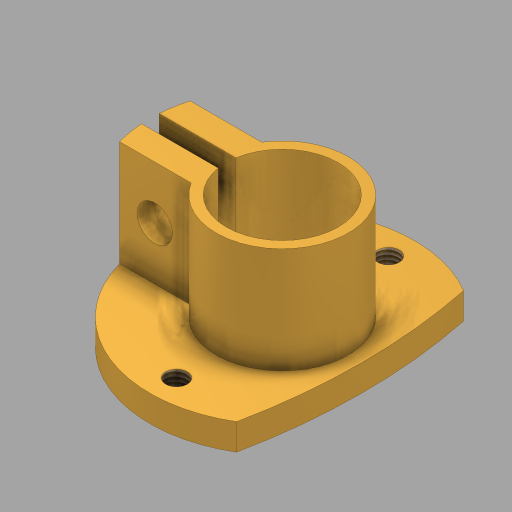
# Autodesk Inventor part: BaffleClampWithScrew
Saved by Autodesk Inventor 2024 (Build 280153020, 153B)
## iProperties
Created: 2023-10-26
Part Number: BaffleClampWithScrew
Material: Brass, Soft Yellow
Document SubType Name: Modeling
Designer: schanen
Density: 8.47 g/cm^3
Appearance: Brass - Satin
Mass: 5.52616 g
Surface Area: 9.72882 cm^2
Volume: 0.652439 cm^3
Author: schanen
Autodesk Inventor part; units mm, degrees
ref_plane "YZ Plane" through (0, 0, 0) normal (1, 0, 0) x (0, 1, 0)
ref_plane "XZ Plane" through (0, 0, 0) normal (0, 1, 0) x (-1, 0, 0)
ref_plane "XY Plane" through (0, 0, 0) normal (0, 0, 1) x (1, 0, 0)
sketch "Sketch1" plane through (0, 0, 0) normal (0, 0, 1) x (1, 0, 0)
  line L0 (-15, 0) -> (-6.35, 0)
  line L1 (-6.35, 0) -> (-6.35, 15)
  line L2 (-6.35, 15) -> (-7.5, 15)
  line L3 (-7.5, 15) -> (-7.5, 3)
  line L4 (-7.5, 3) -> (-15, 3)
  line L5 (-15, 3) -> (-15, 0)
  line L6 (0, -3) -> (0, 18) projected
  point P0 (0, 0)
  dimension "d0" = 3
  dimension "d2" = 15
  dimension "d3" = 6.35
  dimension "d4" = 15
  dimension "d17" = 7.5
  dimension "d18" = 1.15
  constraints: 12 end point, 4 perpendicular, 1 horizontal, 1 horizontal alignment, 1 parallel
  measures "d0" distance of L4.end L0.start
  measures "d2" distance of L0.end L1.end
  measures "d3" distance from line of point (0, 0) L1
  measures "d4" distance from line of point (0, 0) L5
  measures "d17" distance between parallel lines of L6 L3
  measures "d18" distance between parallel lines of L1 L3
revolve "Revolution1" add sketch "Sketch1" angle 360 about axis through (0, -10, 0) along (0, 1, 0)
sketch "Sketch2" plane through (0, 3, 0) normal (0, 1, 0) x (1, 0, 0)
  point P0 (0, 0)
  point P1 (0.0472, 12)
  point P2 (0, -12)
  dimension "d6" = 12
  dimension "d22" = 12
  measures "d6" vertical distance of point (0, 0) point (0.047, 12)
  measures "d22" distance of point (0, 0) point (0, -12)
hole "Hole1" at (0.0472, 3, -12) at (0, 3, 12) direction (0, -1, 0) diameter 2.459 end through all thread size "M3x0.5" class "6H" standard "ISO Metric profile"
sketch "Sketch4" plane through (0, 3, 0) normal (0, 1, 0) x (1, 0, 0)
  circle A0 centre (0, 0) radius 15 projected
  circle A1 centre (0, 0) radius 7.5 projected
  circle A2 centre (-55, 0) radius 64
  point P0 (7.6909, 12.8783)
  point P1 (7.5, 0)
  point P2 (7.6909, -12.8783)
  dimension "d23" = 128
  dimension "d24" = 55
  constraints: 1 centre point, 1 horizontal alignment
  measures "d23" diameter of A2
  measures "d24" distance of A2.centre point (0, 0)
extrude "Extrusion2" cut sketch "Sketch4" against normal through all contours A0 A2 picked at (10.8452, -2.4648)
sketch "Sketch6" plane through (0, 3, 0) normal (0, 1, 0) x (1, 0, 0)
  arc A0 (7.6909, 12.8783) -> (7.6909, -12.8783) centre (0, 0) ccw projected
  circle A1 centre (0, 0) radius 7.5 projected
  line L0 (-6.3443, 4) -> (-15, 4)
  line L1 (-15, 4) -> (-15, -4)
  line L2 (-15, -4) -> (-6.3443, -4)
  line L3 (-6.3443, -4) -> (-6.3443, 4)
  point P0 (-14.4568, -4)
  point P1 (-6.3443, -4)
  point P2 (-14.4568, 4)
  dimension "d32" = 4
  dimension "d33" = 4
  constraints: 8 end point, 2 parallel, 1 horizontal, 1 perpendicular, 2 other
  measures "d32" distance from line of point (0, 0) L2
  measures "d33" distance from line of point (0, 0) L0
extrude "Extrusion3" add sketch "Sketch6" along normal up to surface (12 mm away) contours L0 A1 L2 A0
sketch "Sketch7" plane through (-14.4568, 15, -4) normal (0, 1, 0) x (1, 0, 0)
  circle A0 centre (14.4568, -4) radius 6.35 projected
  line L0 (8.1861, -5) -> (-0.5432, -5)
  line L1 (-0.5432, -5) -> (-0.5432, -3)
  line L2 (-0.5432, -3) -> (8.1861, -3)
  line L3 (8.1861, -3) -> (8.1861, -5)
  arc A1 (0, 0) -> (0, -8) centre (14.4568, -4) ccw projected
  point P0 (-0.5098, -5)
  point P1 (8.1861, -3)
  point P2 (-0.5098, -3)
  dimension "d27" = 1
  dimension "d28" = 1
  constraints: 8 end point, 2 parallel, 1 horizontal, 1 perpendicular, 1 tangent, 2 other
  measures "d27" distance from line of point (14.457, -4) L0
  measures "d28" distance from line of point (14.457, -4) L2
extrude "Extrusion4" cut sketch "Sketch7" against normal through all contours A0 L0 A1 L2
sketch "Sketch8" plane through (-14.4568, 3, 4) normal (0, 0, 1) x (1, 0, 0)
  line L0 (0, 0) -> (0, 12) projected
  line L1 (8.1125, 12) -> (0, 12) projected
  point P0 (7.0914, 12)
  point P1 (4, 6)
  dimension "d35" = 12
  dimension "d37" = 4
  dimension "d38" = 6
  measures "d35" distance of L0.start L0.end
  measures "d37" distance from line of L0 point (4, 6)
  measures "d38" distance from line of L1 point (4, 6)
hole "Hole2" at (-10.4568, 9, 4) direction (0, 0, -1) diameter 4 end through all
equation "\"d22\" = d6"
equation "\"d24\" = tubes_r"
equation "\"d33\" = d32"
equation "\"d28\" = d27"
equation "\"d38\" = 0.5 * d35"
equation "\"tubes_r\" = 55"
body "Solid1"
